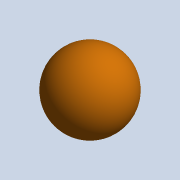
# Autodesk Inventor part: Golfball
Saved by Autodesk Inventor 2021 (Build 250183000, 183)
## iProperties
Part Number: Golfball
Material: ABS-Kunststoff
Document SubType Name: Modellieren
Designer: Timo de Vries
Appearance: Glatt - Weiß
Mass: 43.1194 g
Surface Area: 57.1999 cm^2
Volume: 40.6787 cm^3
Density: 1.06 g/cm^3
Author: Timo de Vries
Autodesk Inventor part; units mm, degrees
ref_plane "YZ-Ebene" through (0, 0, 0) normal (1, 0, 0) x (0, 1, 0)
ref_plane "XZ-Ebene" through (0, 0, 0) normal (0, 1, 0) x (-1, 0, 0)
ref_plane "XY-Ebene" through (0, 0, 0) normal (0, 0, 1) x (1, 0, 0)
sketch "Skizze2" plane through (0, 0, 0) normal (0, 0, 1) x (1, 0, 0)
  arc A0 (21.335, 0) -> (-21.335, 0) centre (0, 0) ccw
  line L0 (-21.335, 0) -> (21.335, 0)
  dimension "d1" = 21.335
  constraints: 2 coincident, 2 end point, 2 point on circle, 1 centre point, 1 horizontal, 1 midpoint
  measures "d1" radius of A0
revolve "Umdrehung1" add sketch "Skizze2" angle 360 about axis through (-21.335, 0, 0) along (1, 0, 0)
